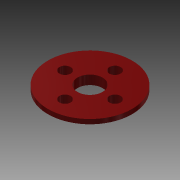
# Autodesk Inventor part: arm_coupler2
Saved by Autodesk Inventor 2013 (Build 170138000, 138)
## iProperties
Created: 2014-10-25
Part Number: arm_coupler2
Material: ABS Plastic
Document SubType Name: Modeling
Designer: Masta
Density: 1 g/cm^3
Author: Masta
Autodesk Inventor part; units mm, degrees
ref_plane "YZ Plane" through (0, 0, 0) normal (1, 0, 0) x (0, 1, 0)
ref_plane "XZ Plane" through (0, 0, 0) normal (0, 1, 0) x (-1, 0, 0)
ref_plane "XY Plane" through (0, 0, 0) normal (0, 0, 1) x (1, 0, 0)
sketch "Sketch1" plane through (0, 0, 0) normal (0, 0, 1) x (1, 0, 0)
  circle A0 centre (0, 0) radius 14
  circle A1 centre (0, 0) radius 18.5
  line L0 (0, 0) -> (11, 0) construction
  dimension "d0" = 28
  dimension "d1" = 37
  dimension "d6" = 11
  constraints: 3 coincident, 2 centre point, 2 end point, 1 horizontal
  measures "d0" diameter of A0
  measures "d1" diameter of A1
  measures "d6" distance of L0.start L0.end
extrude "Extrusion1" add sketch "Sketch1" against normal blind 2 contours A0 | A1
extrude "Extrusion2" add sketch "Sketch1" against normal blind 4 contours A0
hole "Hole1" at (11, 0, 0) direction (0, 0, -1) diameter 5 end through all
pattern_circular "Circular Pattern1" count 4 over 360 about axis through (0, 0, -10) along (0, 0, 1) of "Hole1"
hole "Hole2" at (0, 0, 0) direction (0, 0, -1) diameter 11 end through all
body "Solid1"
